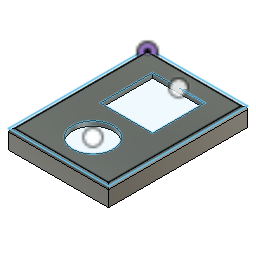
TopSnake (Autodesk Fusion 360 design; units mm, degrees)
Autodesk Fusion 360 part; units mm, degrees
sketch "Sketch1" plane through (0, 0, 0) normal (0, 0, 1) x (1, 0, 0)
  line L0 (0, 0) -> (60, 0)
  line L1 (0, 0) -> (0, -85)
  line L2 (0, -85) -> (60, -85)
  line L3 (60, -85) -> (60, 0)
  line L4 (30, -10) -> (46.75, -10)
  line L5 (46.75, -10) -> (13.25, -10)
  line L6 (13.25, -10) -> (13.25, -43.5)
  line L7 (13.25, -43.5) -> (46.75, -43.5)
  line L8 (46.75, -43.5) -> (46.75, -10)
  circle A0 centre (30, -65) radius 13
  line L9 (62, -87) -> (-2, -87)
  line L10 (-2, -87) -> (-2, 2)
  line L11 (-2, 2) -> (62, 2)
  line L12 (62, 2) -> (62, -87)
  dimension "d1" = 60
  dimension "d2" = 85
  dimension "d3" = 60
  dimension "d4" = 16.75
  dimension "d5" = 33.5
  dimension "d6" = 33.5
  dimension "d7" = 33.5
  dimension "d8" = 26
  constraint horizontal L0
  constraint coincident L0.start L1.start
  constraint perpendicular L0 L1
  constraint perpendicular L1 L2
  constraint perpendicular L1 L4
  constraint perpendicular L1 L5
  constraint perpendicular L5 L6
  constraint perpendicular L6 L7
  constraint horizontal L9
  constraint vertical L10
  constraint horizontal L11
  constraint vertical L12
  measures "d1" distance of L0.start L0.end
  measures "d2" distance of L0.start L1.end
  measures "d3" distance of L1.end L2.end
  measures "d4" distance of L4.start L4.end
  measures "d5" distance of L4.end L5.end
  measures "d6" distance of L5.end L6.end
  measures "d7" distance of L6.end L7.end
  measures "d8" diameter of A0
extrude "Extrude1" add sketch "Sketch1" against normal blind 3 contours L0 L1 L2 L3 | L9 L10 L11 L12
extrude "Extrude2" add sketch "Sketch1" against normal blind 12 contours L9 L10 L11 L12
fillet "Fillet1" radius 2 4 edges at (-2, -42.5, 0) (30, 2, 0) (62, -42.5, 0) (30, -87, 0)
